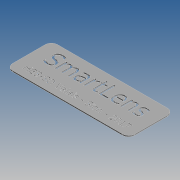
# Autodesk Inventor part: P306PlaqueLogo
Saved by Autodesk Inventor 2015 SP1 (Build 190203100, 203)
## iProperties
Created: 2017-01-31
Part Number: P306PlaqueLogo
Material: Générique
Document SubType Name: Modeling
Designer: serge.amoos
Density: 1 g/cm^3
Appearance: Par défaut
Author: serge.amoos
Autodesk Inventor part; units mm, degrees
ref_plane "YZ Plane" through (0, 0, 0) normal (1, 0, 0) x (0, 1, 0)
ref_plane "XZ Plane" through (0, 0, 0) normal (0, 1, 0) x (-1, 0, 0)
ref_plane "XY Plane" through (0, 0, 0) normal (0, 0, 1) x (1, 0, 0)
sketch "Sketch1" plane through (0, 0, 0) normal (0, 0, 1) x (1, 0, 0)
  line L0 (-27.65, 0) -> (27.65, 0) construction
  line L1 (0, -10.15) -> (0, 10.15) construction
  line L2 (-19.75, 7.25) -> (19.75, 7.25)
  line L3 (19.75, 7.25) -> (19.75, -7.25)
  line L4 (19.75, -7.25) -> (-19.75, -7.25)
  line L5 (-19.75, -7.25) -> (-19.75, 7.25)
  point P0 (0, 0)
  point P1 (0, 7.25)
  point P2 (19.75, 0)
  dimension "d0" = 39.5
  dimension "d1" = 14.5
  constraints: 8 end point, 2 midpoint, 2 parallel, 2 point on line, 1 horizontal, 1 perpendicular
  measures "d0" distance of L2.start L2.end
  measures "d1" distance of L2.end L3.end
extrude "Extrusion1" add sketch "Sketch1" along normal blind 0.4
fillet "Fillet1" radius 2 4 edges at (19.75, -7.25, 0.2) (19.75, 7.25, 0.2) (-19.75, 7.25, 0.2) (-19.75, -7.25, 0.2)
sketch "Sketch2" plane through (0, 0, 0.4) normal (0, 0, 1) x (1, 0, 0)
  line L0 (-29.6663, 8.3891) -> (29.6663, 8.3891) construction
  line L1 (29.6663, 8.3891) -> (29.6663, -8.3891) construction
  line L2 (29.6663, -8.3891) -> (-29.6663, -8.3891) construction
  line L3 (-29.6663, -8.3891) -> (-29.6663, 8.3891) construction
  line L4 (19.75, -5.25) -> (19.75, 5.25) projected
  line L5 (17.75, 7.25) -> (-17.75, 7.25) projected
  spline S0 degree 2 poles (-14.066, 0.0243) (-14.609, 0.0243) (-15.3707, 0.2512) (-15.707, 0.4133) knots 0 0 0 1 2 2 2
  line L6 (-15.707, 0.4133) -> (-15.707, 1.248)
  line L7 (-15.707, 1.248) -> (-15.6584, 1.248)
  spline S1 degree 2 poles (-15.6584, 1.248) (-15.3302, 0.94) (-14.4996, 0.5997) (-14.1147, 0.5997) knots 0 0 0 1 2 2 2
  spline S2 degree 2 poles (-14.1147, 0.5997) (-13.5636, 0.5997) (-13.0004, 1.0575) (-13.0004, 1.4343) knots 0 0 0 1 2 2 2
  spline S3 degree 2 poles (-13.0004, 1.4343) (-13.0004, 1.7342) (-13.2962, 2.1069) (-13.6163, 2.2001) knots 0 0 0 1 2 2 2
  spline S4 degree 2 poles (-13.6163, 2.2001) (-13.8472, 2.265) (-14.2322, 2.3541) (-14.5199, 2.427) knots 0 0 0 1 2 2 2
  spline S5 degree 2 poles (-14.5199, 2.427) (-14.7792, 2.4959) (-15.1884, 2.7026) (-15.3464, 2.8687) knots 0 0 0 1 2 2 2
  spline S6 degree 2 poles (-15.3464, 2.8687) (-15.5004, 3.0348) (-15.6706, 3.4805) (-15.6706, 3.7723) knots 0 0 0 1 2 2 2
  spline S7 degree 2 poles (-15.6706, 3.7723) (-15.6706, 4.38) (-14.7224, 5.2026) (-13.9891, 5.2026) knots 0 0 0 1 2 2 2
  spline S8 degree 2 poles (-13.9891, 5.2026) (-13.5677, 5.2026) (-12.8221, 5.0364) (-12.502, 4.8784) knots 0 0 0 1 2 2 2
  line L8 (-12.502, 4.8784) -> (-12.502, 4.0843)
  line L9 (-12.502, 4.0843) -> (-12.5506, 4.0843)
  spline S9 degree 2 poles (-12.5506, 4.0843) (-12.7897, 4.3031) (-13.5353, 4.6272) (-13.9445, 4.6272) knots 0 0 0 1 2 2 2
  spline S10 degree 2 poles (-13.9445, 4.6272) (-14.4064, 4.6272) (-14.9777, 4.1937) (-14.9777, 3.8411) knots 0 0 0 1 2 2 2
  spline S11 degree 2 poles (-14.9777, 3.8411) (-14.9777, 3.5251) (-14.6414, 3.1483) (-14.3254, 3.0632) knots 0 0 0 1 2 2 2
  spline S12 degree 2 poles (-14.3254, 3.0632) (-14.1147, 3.0065) (-13.5028, 2.8606) (-13.3002, 2.7998) knots 0 0 0 1 2 2 2
  spline S13 degree 2 poles (-13.3002, 2.7998) (-12.7857, 2.6418) (-12.3075, 2.0057) (-12.3075, 1.5397) knots 0 0 0 1 2 2 2
  spline S14 degree 2 poles (-12.3075, 1.5397) (-12.3075, 1.2439) (-12.5466, 0.6766) (-12.7613, 0.4781) knots 0 0 0 1 2 2 2
  spline S15 degree 2 poles (-12.7613, 0.4781) (-13.0004, 0.2593) (-13.6082, 0.0243) (-14.066, 0.0243) knots 0 0 0 1 2 2 2
  line L10 (-7.425, 0.1134) -> (-7.425, 2.2852)
  spline S16 degree 2 poles (-7.425, 2.2852) (-7.425, 2.5446) (-7.4656, 2.9862) (-7.5304, 3.1078) knots 0 0 0 1 2 2 2
  spline S17 degree 2 poles (-7.5304, 3.1078) (-7.5952, 3.2415) (-7.8424, 3.3711) (-8.0571, 3.3711) knots 0 0 0 1 2 2 2
  spline S18 degree 2 poles (-8.0571, 3.3711) (-8.2516, 3.3711) (-8.6973, 3.1321) (-8.9323, 2.9052) knots 0 0 0 1 2 2 2
  spline S19 degree 2 poles (-8.9323, 2.9052) (-8.9283, 2.8484) (-8.9202, 2.6904) (-8.9202, 2.5851) knots 0 0 0 1 2 2 2
  line L11 (-8.9202, 2.5851) -> (-8.9202, 0.1134)
  line L12 (-8.9202, 0.1134) -> (-9.5523, 0.1134)
  line L13 (-9.5523, 0.1134) -> (-9.5523, 2.2852)
  spline S20 degree 2 poles (-9.5523, 2.2852) (-9.5523, 2.5446) (-9.5928, 2.9862) (-9.6576, 3.1078) knots 0 0 0 1 2 2 2
  spline S21 degree 2 poles (-9.6576, 3.1078) (-9.7224, 3.2415) (-9.9696, 3.3711) (-10.1844, 3.3711) knots 0 0 0 1 2 2 2
  spline S22 degree 2 poles (-10.1844, 3.3711) (-10.387, 3.3711) (-10.8367, 3.1159) (-11.0474, 2.9173) knots 0 0 0 1 2 2 2
  line L14 (-11.0474, 2.9173) -> (-11.0474, 0.1134)
  line L15 (-11.0474, 0.1134) -> (-11.6795, 0.1134)
  line L16 (-11.6795, 0.1134) -> (-11.6795, 3.8655)
  line L17 (-11.6795, 3.8655) -> (-11.0474, 3.8655)
  line L18 (-11.0474, 3.8655) -> (-11.0474, 3.4522)
  spline S23 degree 2 poles (-11.0474, 3.4522) (-10.8002, 3.6993) (-10.314, 3.9708) (-10.0223, 3.9708) knots 0 0 0 1 2 2 2
  spline S24 degree 2 poles (-10.0223, 3.9708) (-9.69, 3.9708) (-9.1754, 3.6669) (-9.0417, 3.3225) knots 0 0 0 1 2 2 2
  spline S25 degree 2 poles (-9.0417, 3.3225) (-8.7541, 3.6426) (-8.2111, 3.9708) (-7.8951, 3.9708) knots 0 0 0 1 2 2 2
  spline S26 degree 2 poles (-7.8951, 3.9708) (-7.6519, 3.9708) (-7.2549, 3.8209) (-7.109, 3.6507) knots 0 0 0 1 2 2 2
  spline S27 degree 2 poles (-7.109, 3.6507) (-6.9591, 3.4805) (-6.7929, 2.97) (-6.7929, 2.5851) knots 0 0 0 1 2 2 2
  line L19 (-6.7929, 2.5851) -> (-6.7929, 0.1134)
  line L20 (-6.7929, 0.1134) -> (-7.425, 0.1134)
  spline S28 degree 2 poles (-3.8148, 0.5105) (-3.8918, 0.4538) (-4.1511, 0.2512) (-4.2727, 0.1904) knots 0 0 0 1 2 2 2
  spline S29 degree 2 poles (-4.2727, 0.1904) (-4.4388, 0.1013) (-4.7508, 0.0081) (-5.0344, 0.0081) knots 0 0 0 1 2 2 2
  spline S30 degree 2 poles (-5.0344, 0.0081) (-5.2654, 0.0081) (-5.6827, 0.1823) (-5.8408, 0.3403) knots 0 0 0 1 2 2 2
  spline S31 degree 2 poles (-5.8408, 0.3403) (-5.9907, 0.4943) (-6.173, 0.9481) (-6.173, 1.1993) knots 0 0 0 1 2 2 2
  spline S32 degree 2 poles (-6.173, 1.1993) (-6.173, 1.5883) (-5.8448, 2.1394) (-5.4882, 2.2974) knots 0 0 0 1 2 2 2
  spline S33 degree 2 poles (-5.4882, 2.2974) (-5.1722, 2.4433) (-4.3132, 2.5527) (-3.8148, 2.581) knots 0 0 0 1 2 2 2
  line L21 (-3.8148, 2.581) -> (-3.8148, 2.7026)
  spline S34 degree 2 poles (-3.8148, 2.7026) (-3.8148, 2.9214) (-3.9485, 3.1928) (-4.0701, 3.2698) knots 0 0 0 1 2 2 2
  spline S35 degree 2 poles (-4.0701, 3.2698) (-4.1917, 3.3468) (-4.5401, 3.3954) (-4.7265, 3.3954) knots 0 0 0 1 2 2 2
  spline S36 degree 2 poles (-4.7265, 3.3954) (-4.9453, 3.3954) (-5.5369, 3.2658) (-5.8327, 3.1402) knots 0 0 0 1 2 2 2
  line L22 (-5.8327, 3.1402) -> (-5.8691, 3.1402)
  line L23 (-5.8691, 3.1402) -> (-5.8691, 3.7844)
  spline S37 degree 2 poles (-5.8691, 3.7844) (-5.6949, 3.833) (-5.0425, 3.9546) (-4.7224, 3.9546) knots 0 0 0 1 2 2 2
  spline S38 degree 2 poles (-4.7224, 3.9546) (-4.3335, 3.9546) (-3.8027, 3.833) (-3.592, 3.675) knots 0 0 0 1 2 2 2
  spline S39 degree 2 poles (-3.592, 3.675) (-3.3853, 3.5211) (-3.1827, 3.0308) (-3.1827, 2.6783) knots 0 0 0 1 2 2 2
  line L24 (-3.1827, 2.6783) -> (-3.1827, 0.1134)
  line L25 (-3.1827, 0.1134) -> (-3.8148, 0.1134)
  line L26 (-3.8148, 0.1134) -> (-3.8148, 0.5105)
  line L27 (-3.8148, 1.0373) -> (-3.8148, 2.0786)
  spline S40 degree 2 poles (-3.8148, 2.0786) (-4.0417, 2.0583) (-4.7265, 1.9894) (-4.9412, 1.9246) knots 0 0 0 1 2 2 2
  spline S41 degree 2 poles (-4.9412, 1.9246) (-5.1925, 1.8476) (-5.5207, 1.5275) (-5.5207, 1.2439) knots 0 0 0 1 2 2 2
  spline S42 degree 2 poles (-5.5207, 1.2439) (-5.5207, 0.9198) (-5.156, 0.5916) (-4.8075, 0.5916) knots 0 0 0 1 2 2 2
  spline S43 degree 2 poles (-4.8075, 0.5916) (-4.5117, 0.5916) (-4.0255, 0.8468) (-3.8148, 1.0373) knots 0 0 0 1 2 2 2
  line L28 (-0.3059, 3.1888) -> (-0.3383, 3.1888)
  spline S44 degree 2 poles (-0.3383, 3.1888) (-0.4113, 3.2091) (-0.5693, 3.2172) (-0.6787, 3.2172) knots 0 0 0 1 2 2 2
  spline S45 degree 2 poles (-0.6787, 3.2172) (-0.934, 3.2172) (-1.4364, 2.9943) (-1.6633, 2.7755) knots 0 0 0 1 2 2 2
  line L29 (-1.6633, 2.7755) -> (-1.6633, 0.1134)
  line L30 (-1.6633, 0.1134) -> (-2.2954, 0.1134)
  line L31 (-2.2954, 0.1134) -> (-2.2954, 3.8655)
  line L32 (-2.2954, 3.8655) -> (-1.6633, 3.8655)
  line L33 (-1.6633, 3.8655) -> (-1.6633, 3.3063)
  spline S46 degree 2 poles (-1.6633, 3.3063) (-1.3189, 3.6142) (-0.8043, 3.8655) (-0.5612, 3.8655) knots 0 0 0 1 2 2 2
  spline S47 degree 2 poles (-0.5612, 3.8655) (-0.4639, 3.8655) (-0.3667, 3.8574) (-0.3059, 3.8452) knots 0 0 0 1 2 2 2
  line L34 (-0.3059, 3.8452) -> (-0.3059, 3.1888)
  spline S48 degree 2 poles (1.3189, 0.0405) (0.8043, 0.0405) (0.2249, 0.628) (0.2249, 1.2642) knots 0 0 0 1 2 2 2
  line L35 (0.2249, 1.2642) -> (0.2249, 3.3428)
  line L36 (0.2249, 3.3428) -> (-0.2006, 3.3428)
  line L37 (-0.2006, 3.3428) -> (-0.2006, 3.8655)
  line L38 (-0.2006, 3.8655) -> (0.2249, 3.8655)
  line L39 (0.2249, 3.8655) -> (0.2249, 4.9433)
  line L40 (0.2249, 4.9433) -> (0.857, 4.9433)
  line L41 (0.857, 4.9433) -> (0.857, 3.8655)
  line L42 (0.857, 3.8655) -> (2.0199, 3.8655)
  line L43 (2.0199, 3.8655) -> (2.0199, 3.3428)
  line L44 (2.0199, 3.3428) -> (0.857, 3.3428)
  line L45 (0.857, 3.3428) -> (0.857, 1.5559)
  spline S49 degree 2 poles (0.857, 1.5559) (0.857, 1.2723) (0.8772, 0.9603) (0.9461, 0.8266) knots 0 0 0 1 2 2 2
  spline S50 degree 2 poles (0.9461, 0.8266) (1.0028, 0.7091) (1.2581, 0.5916) (1.4769, 0.5916) knots 0 0 0 1 2 2 2
  spline S51 degree 2 poles (1.4769, 0.5916) (1.6309, 0.5916) (1.9186, 0.6847) (1.9834, 0.7131) knots 0 0 0 1 2 2 2
  line L46 (1.9834, 0.7131) -> (2.0199, 0.7131)
  line L47 (2.0199, 0.7131) -> (2.0199, 0.1458)
  spline S52 degree 2 poles (2.0199, 0.1458) (1.8416, 0.0972) (1.4769, 0.0405) (1.3189, 0.0405) knots 0 0 0 1 2 2 2
  line L48 (5.4315, 0.1134) -> (2.5344, 0.1134)
  line L49 (2.5344, 0.1134) -> (2.5344, 5.1134)
  line L50 (2.5344, 5.1134) -> (3.1989, 5.1134)
  line L51 (3.1989, 5.1134) -> (3.1989, 0.705)
  line L52 (3.1989, 0.705) -> (5.4315, 0.705)
  line L53 (5.4315, 0.705) -> (5.4315, 0.1134)
  spline S53 degree 2 poles (7.5344, 0.0283) (6.6349, 0.0283) (5.6463, 1.0373) (5.6463, 1.9692) knots 0 0 0 1 2 2 2
  spline S54 degree 2 poles (5.6463, 1.9692) (5.6463, 2.8849) (6.6066, 3.9708) (7.3805, 3.9708) knots 0 0 0 1 2 2 2
  spline S55 degree 2 poles (7.3805, 3.9708) (7.7289, 3.9708) (8.2678, 3.7682) (8.4664, 3.5535) knots 0 0 0 1 2 2 2
  spline S56 degree 2 poles (8.4664, 3.5535) (8.669, 3.3387) (8.8837, 2.7188) (8.8837, 2.269) knots 0 0 0 1 2 2 2
  line L54 (8.8837, 2.269) -> (8.8837, 1.9246)
  line L55 (8.8837, 1.9246) -> (6.2865, 1.9246)
  spline S57 degree 2 poles (6.2865, 1.9246) (6.2865, 1.2723) (6.9429, 0.5794) (7.5263, 0.5794) knots 0 0 0 1 2 2 2
  spline S58 degree 2 poles (7.5263, 0.5794) (7.733, 0.5794) (8.1341, 0.6726) (8.2962, 0.7455) knots 0 0 0 1 2 2 2
  spline S59 degree 2 poles (8.2962, 0.7455) (8.4664, 0.8266) (8.7014, 0.9684) (8.7784, 1.0332) knots 0 0 0 1 2 2 2
  line L56 (8.7784, 1.0332) -> (8.8148, 1.0332)
  line L57 (8.8148, 1.0332) -> (8.8148, 0.3444)
  spline S60 degree 2 poles (8.8148, 0.3444) (8.7054, 0.2998) (8.3732, 0.1702) (8.2435, 0.1337) knots 0 0 0 1 2 2 2
  spline S61 degree 2 poles (8.2435, 0.1337) (8.0612, 0.081) (7.7613, 0.0283) (7.5344, 0.0283) knots 0 0 0 1 2 2 2
  spline S62 degree 2 poles (8.2678, 2.4068) (8.2597, 2.6621) (8.1544, 3.0348) (8.0531, 3.1604) knots 0 0 0 1 2 2 2
  spline S63 degree 2 poles (8.0531, 3.1604) (7.9437, 3.3022) (7.5993, 3.4522) (7.344, 3.4522) knots 0 0 0 1 2 2 2
  spline S64 degree 2 poles (7.344, 3.4522) (7.0928, 3.4522) (6.7403, 3.3022) (6.5944, 3.1564) knots 0 0 0 1 2 2 2
  spline S65 degree 2 poles (6.5944, 3.1564) (6.4526, 3.0065) (6.3067, 2.6458) (6.2865, 2.4068) knots 0 0 0 1 2 2 2
  line L58 (6.2865, 2.4068) -> (8.2678, 2.4068)
  line L59 (12.4696, 0.1134) -> (11.8375, 0.1134)
  line L60 (11.8375, 0.1134) -> (11.8375, 2.2528)
  spline S66 degree 2 poles (11.8375, 2.2528) (11.8375, 2.5121) (11.7889, 2.9578) (11.716, 3.0916) knots 0 0 0 1 2 2 2
  spline S67 degree 2 poles (11.716, 3.0916) (11.639, 3.2334) (11.3635, 3.3711) (11.1284, 3.3711) knots 0 0 0 1 2 2 2
  spline S68 degree 2 poles (11.1284, 3.3711) (10.8934, 3.3711) (10.3951, 3.1199) (10.156, 2.9173) knots 0 0 0 1 2 2 2
  line L61 (10.156, 2.9173) -> (10.156, 0.1134)
  line L62 (10.156, 0.1134) -> (9.5239, 0.1134)
  line L63 (9.5239, 0.1134) -> (9.5239, 3.8655)
  line L64 (9.5239, 3.8655) -> (10.156, 3.8655)
  line L65 (10.156, 3.8655) -> (10.156, 3.4481)
  spline S69 degree 2 poles (10.156, 3.4481) (10.4396, 3.7034) (10.9866, 3.9708) (11.2946, 3.9708) knots 0 0 0 1 2 2 2
  spline S70 degree 2 poles (11.2946, 3.9708) (11.8456, 3.9708) (12.4696, 3.2415) (12.4696, 2.5486) knots 0 0 0 1 2 2 2
  line L66 (12.4696, 2.5486) -> (12.4696, 0.1134)
  spline S71 degree 2 poles (14.3699, 0.0243) (13.9931, 0.0243) (13.3408, 0.2269) (13.126, 0.3403) knots 0 0 0 1 2 2 2
  line L67 (13.126, 0.3403) -> (13.126, 1.0494)
  line L68 (13.126, 1.0494) -> (13.1584, 1.0494)
  spline S72 degree 2 poles (13.1584, 1.0494) (13.2395, 0.9846) (13.4583, 0.8306) (13.6406, 0.7455) knots 0 0 0 1 2 2 2
  spline S73 degree 2 poles (13.6406, 0.7455) (13.7986, 0.6685) (14.1876, 0.5551) (14.3942, 0.5551) knots 0 0 0 1 2 2 2
  spline S74 degree 2 poles (14.3942, 0.5551) (14.5442, 0.5551) (14.8886, 0.624) (14.9696, 0.6807) knots 0 0 0 1 2 2 2
  spline S75 degree 2 poles (14.9696, 0.6807) (15.0871, 0.7577) (15.1925, 0.9319) (15.1925, 1.1102) knots 0 0 0 1 2 2 2
  spline S76 degree 2 poles (15.1925, 1.1102) (15.1925, 1.333) (14.9494, 1.564) (14.6374, 1.641) knots 0 0 0 1 2 2 2
  spline S77 degree 2 poles (14.6374, 1.641) (14.5158, 1.6693) (14.1268, 1.7504) (13.9607, 1.795) knots 0 0 0 1 2 2 2
  spline S78 degree 2 poles (13.9607, 1.795) (13.5312, 1.9206) (13.1422, 2.4392) (13.1422, 2.8079) knots 0 0 0 1 2 2 2
  spline S79 degree 2 poles (13.1422, 2.8079) (13.1422, 3.3185) (13.908, 3.9546) (14.5401, 3.9546) knots 0 0 0 1 2 2 2
  spline S80 degree 2 poles (14.5401, 3.9546) (14.8521, 3.9546) (15.4842, 3.8006) (15.6989, 3.6831) knots 0 0 0 1 2 2 2
  line L69 (15.6989, 3.6831) -> (15.6989, 3.0065)
  line L70 (15.6989, 3.0065) -> (15.6665, 3.0065)
  spline S81 degree 2 poles (15.6665, 3.0065) (15.4234, 3.201) (14.8318, 3.4238) (14.528, 3.4238) knots 0 0 0 1 2 2 2
  spline S82 degree 2 poles (14.528, 3.4238) (14.216, 3.4238) (13.7865, 3.1604) (13.7865, 2.8971) knots 0 0 0 1 2 2 2
  spline S83 degree 2 poles (13.7865, 2.8971) (13.7865, 2.658) (14.0417, 2.427) (14.3254, 2.3541) knots 0 0 0 1 2 2 2
  spline S84 degree 2 poles (14.3254, 2.3541) (14.4631, 2.3176) (14.8116, 2.2447) (15.002, 2.2001) knots 0 0 0 1 2 2 2
  spline S85 degree 2 poles (15.002, 2.2001) (15.4153, 2.0948) (15.8367, 1.6126) (15.8367, 1.1953) knots 0 0 0 1 2 2 2
  spline S86 degree 2 poles (15.8367, 1.1953) (15.8367, 0.9522) (15.6463, 0.5227) (15.4599, 0.3646) knots 0 0 0 1 2 2 2
  spline S87 degree 2 poles (15.4599, 0.3646) (15.2613, 0.1985) (14.7549, 0.0243) (14.3699, 0.0243) knots 0 0 0 1 2 2 2
  line L71 (-15.2974, -5.1604) -> (-15.5632, -5.1604)
  line L72 (-15.5632, -5.1604) -> (-15.5632, -4.1815)
  line L73 (-15.5632, -4.1815) -> (-16.4838, -4.1815)
  line L74 (-16.4838, -4.1815) -> (-16.4838, -5.1604)
  line L75 (-16.4838, -5.1604) -> (-16.7496, -5.1604)
  line L76 (-16.7496, -5.1604) -> (-16.7496, -3.1604)
  line L77 (-16.7496, -3.1604) -> (-16.4838, -3.1604)
  line L78 (-16.4838, -3.1604) -> (-16.4838, -3.9449)
  line L79 (-16.4838, -3.9449) -> (-15.5632, -3.9449)
  line L80 (-15.5632, -3.9449) -> (-15.5632, -3.1604)
  line L81 (-15.5632, -3.1604) -> (-15.2974, -3.1604)
  line L82 (-15.2974, -3.1604) -> (-15.2974, -5.1604)
  line L83 (-14.8922, -5.1604) -> (-14.8922, -3.1604)
  line L84 (-14.8922, -3.1604) -> (-13.641, -3.1604)
  line L85 (-13.641, -3.1604) -> (-13.641, -3.3971)
  line L86 (-13.641, -3.3971) -> (-14.6264, -3.3971)
  line L87 (-14.6264, -3.3971) -> (-14.6264, -3.9449)
  line L88 (-14.6264, -3.9449) -> (-13.7075, -3.9449)
  line L89 (-13.7075, -3.9449) -> (-13.7075, -4.1815)
  line L90 (-13.7075, -4.1815) -> (-14.6264, -4.1815)
  line L91 (-14.6264, -4.1815) -> (-14.6264, -4.9238)
  line L92 (-14.6264, -4.9238) -> (-13.641, -4.9238)
  line L93 (-13.641, -4.9238) -> (-13.641, -5.1604)
  line L94 (-13.641, -5.1604) -> (-14.8922, -5.1604)
  spline S88 degree 2 poles (-12.7917, -5.1961) (-13.0089, -5.1961) (-13.3136, -5.1053) (-13.4481, -5.0405) knots 0 0 0 1 2 2 2
  line L95 (-13.4481, -5.0405) -> (-13.4481, -4.7066)
  line L96 (-13.4481, -4.7066) -> (-13.4287, -4.7066)
  spline S89 degree 2 poles (-13.4287, -4.7066) (-13.2974, -4.8298) (-12.9652, -4.9659) (-12.8112, -4.9659) knots 0 0 0 1 2 2 2
  spline S90 degree 2 poles (-12.8112, -4.9659) (-12.5908, -4.9659) (-12.3655, -4.7828) (-12.3655, -4.6321) knots 0 0 0 1 2 2 2
  spline S91 degree 2 poles (-12.3655, -4.6321) (-12.3655, -4.5121) (-12.4838, -4.363) (-12.6118, -4.3258) knots 0 0 0 1 2 2 2
  spline S92 degree 2 poles (-12.6118, -4.3258) (-12.7042, -4.2998) (-12.8582, -4.2642) (-12.9733, -4.235) knots 0 0 0 1 2 2 2
  spline S93 degree 2 poles (-12.9733, -4.235) (-13.077, -4.2074) (-13.2407, -4.1248) (-13.3039, -4.0583) knots 0 0 0 1 2 2 2
  spline S94 degree 2 poles (-13.3039, -4.0583) (-13.3655, -3.9919) (-13.4336, -3.8136) (-13.4336, -3.6969) knots 0 0 0 1 2 2 2
  spline S95 degree 2 poles (-13.4336, -3.6969) (-13.4336, -3.4538) (-13.0543, -3.1248) (-12.7609, -3.1248) knots 0 0 0 1 2 2 2
  spline S96 degree 2 poles (-12.7609, -3.1248) (-12.5924, -3.1248) (-12.2942, -3.1912) (-12.1661, -3.2544) knots 0 0 0 1 2 2 2
  line L97 (-12.1661, -3.2544) -> (-12.1661, -3.5721)
  line L98 (-12.1661, -3.5721) -> (-12.1856, -3.5721)
  spline S97 degree 2 poles (-12.1856, -3.5721) (-12.2812, -3.4846) (-12.5794, -3.3549) (-12.7431, -3.3549) knots 0 0 0 1 2 2 2
  spline S98 degree 2 poles (-12.7431, -3.3549) (-12.9279, -3.3549) (-13.1564, -3.5283) (-13.1564, -3.6693) knots 0 0 0 1 2 2 2
  spline S99 degree 2 poles (-13.1564, -3.6693) (-13.1564, -3.7958) (-13.0219, -3.9465) (-12.8955, -3.9805) knots 0 0 0 1 2 2 2
  spline S100 degree 2 poles (-12.8955, -3.9805) (-12.8112, -4.0032) (-12.5665, -4.0616) (-12.4854, -4.0859) knots 0 0 0 1 2 2 2
  spline S101 degree 2 poles (-12.4854, -4.0859) (-12.2796, -4.1491) (-12.0883, -4.4035) (-12.0883, -4.5899) knots 0 0 0 1 2 2 2
  spline S102 degree 2 poles (-12.0883, -4.5899) (-12.0883, -4.7082) (-12.184, -4.9352) (-12.2699, -5.0146) knots 0 0 0 1 2 2 2
  spline S103 degree 2 poles (-12.2699, -5.0146) (-12.3655, -5.1021) (-12.6086, -5.1961) (-12.7917, -5.1961) knots 0 0 0 1 2 2 2
  line L99 (-11.1418, -4.4068) -> (-11.8987, -4.4068)
  line L100 (-11.8987, -4.4068) -> (-11.8987, -4.1637)
  line L101 (-11.8987, -4.1637) -> (-11.1418, -4.1637)
  line L102 (-11.1418, -4.1637) -> (-11.1418, -4.4068)
  spline S104 degree 2 poles (-10.2618, -5.1961) (-10.4789, -5.1961) (-10.7836, -5.1053) (-10.9182, -5.0405) knots 0 0 0 1 2 2 2
  line L103 (-10.9182, -5.0405) -> (-10.9182, -4.7066)
  line L104 (-10.9182, -4.7066) -> (-10.8987, -4.7066)
  spline S105 degree 2 poles (-10.8987, -4.7066) (-10.7674, -4.8298) (-10.4352, -4.9659) (-10.2812, -4.9659) knots 0 0 0 1 2 2 2
  spline S106 degree 2 poles (-10.2812, -4.9659) (-10.0608, -4.9659) (-9.8355, -4.7828) (-9.8355, -4.6321) knots 0 0 0 1 2 2 2
  spline S107 degree 2 poles (-9.8355, -4.6321) (-9.8355, -4.5121) (-9.9538, -4.363) (-10.0818, -4.3258) knots 0 0 0 1 2 2 2
  spline S108 degree 2 poles (-10.0818, -4.3258) (-10.1742, -4.2998) (-10.3282, -4.2642) (-10.4433, -4.235) knots 0 0 0 1 2 2 2
  spline S109 degree 2 poles (-10.4433, -4.235) (-10.547, -4.2074) (-10.7107, -4.1248) (-10.7739, -4.0583) knots 0 0 0 1 2 2 2
  spline S110 degree 2 poles (-10.7739, -4.0583) (-10.8355, -3.9919) (-10.9036, -3.8136) (-10.9036, -3.6969) knots 0 0 0 1 2 2 2
  spline S111 degree 2 poles (-10.9036, -3.6969) (-10.9036, -3.4538) (-10.5243, -3.1248) (-10.231, -3.1248) knots 0 0 0 1 2 2 2
  spline S112 degree 2 poles (-10.231, -3.1248) (-10.0624, -3.1248) (-9.7642, -3.1912) (-9.6361, -3.2544) knots 0 0 0 1 2 2 2
  line L105 (-9.6361, -3.2544) -> (-9.6361, -3.5721)
  line L106 (-9.6361, -3.5721) -> (-9.6556, -3.5721)
  spline S113 degree 2 poles (-9.6556, -3.5721) (-9.7512, -3.4846) (-10.0494, -3.3549) (-10.2131, -3.3549) knots 0 0 0 1 2 2 2
  spline S114 degree 2 poles (-10.2131, -3.3549) (-10.3979, -3.3549) (-10.6264, -3.5283) (-10.6264, -3.6693) knots 0 0 0 1 2 2 2
  spline S115 degree 2 poles (-10.6264, -3.6693) (-10.6264, -3.7958) (-10.4919, -3.9465) (-10.3655, -3.9805) knots 0 0 0 1 2 2 2
  spline S116 degree 2 poles (-10.3655, -3.9805) (-10.2812, -4.0032) (-10.0365, -4.0616) (-9.9554, -4.0859) knots 0 0 0 1 2 2 2
  spline S117 degree 2 poles (-9.9554, -4.0859) (-9.7496, -4.1491) (-9.5583, -4.4035) (-9.5583, -4.5899) knots 0 0 0 1 2 2 2
  spline S118 degree 2 poles (-9.5583, -4.5899) (-9.5583, -4.7082) (-9.654, -4.9352) (-9.7399, -5.0146) knots 0 0 0 1 2 2 2
  spline S119 degree 2 poles (-9.7399, -5.0146) (-9.8355, -5.1021) (-10.0786, -5.1961) (-10.2618, -5.1961) knots 0 0 0 1 2 2 2
  spline S120 degree 2 poles (-7.8728, -3.389) (-7.7593, -3.5219) (-7.6329, -3.9108) (-7.6329, -4.1604) knots 0 0 0 1 2 2 2
  spline S121 degree 2 poles (-7.6329, -4.1604) (-7.6329, -4.4035) (-7.7561, -4.7974) (-7.8728, -4.9303) knots 0 0 0 1 2 2 2
  spline S122 degree 2 poles (-7.8728, -4.9303) (-7.9959, -5.0697) (-8.3217, -5.2026) (-8.5178, -5.2026) knots 0 0 0 1 2 2 2
  spline S123 degree 2 poles (-8.5178, -5.2026) (-8.7204, -5.2026) (-9.0446, -5.0648) (-9.1629, -4.9303) knots 0 0 0 1 2 2 2
  spline S124 degree 2 poles (-9.1629, -4.9303) (-9.278, -4.7974) (-9.4011, -4.4068) (-9.4011, -4.1604) knots 0 0 0 1 2 2 2
  spline S125 degree 2 poles (-9.4011, -4.1604) (-9.4011, -3.9092) (-9.2763, -3.5267) (-9.1613, -3.389) knots 0 0 0 1 2 2 2
  spline S126 degree 2 poles (-9.1613, -3.389) (-9.0446, -3.2561) (-8.7188, -3.1183) (-8.5178, -3.1183) knots 0 0 0 1 2 2 2
  spline S127 degree 2 poles (-8.5178, -3.1183) (-8.3136, -3.1183) (-7.9862, -3.2609) (-7.8728, -3.389) knots 0 0 0 1 2 2 2
  spline S128 degree 2 poles (-7.91, -4.1604) (-7.91, -3.9627) (-7.9959, -3.6564) (-8.0737, -3.5559) knots 0 0 0 1 2 2 2
  spline S129 degree 2 poles (-8.0737, -3.5559) (-8.1532, -3.4522) (-8.3768, -3.3484) (-8.5162, -3.3484) knots 0 0 0 1 2 2 2
  spline S130 degree 2 poles (-8.5162, -3.3484) (-8.6605, -3.3484) (-8.8776, -3.4489) (-8.9603, -3.5559) knots 0 0 0 1 2 2 2
  spline S131 degree 2 poles (-8.9603, -3.5559) (-9.0397, -3.658) (-9.124, -3.9659) (-9.124, -4.1604) knots 0 0 0 1 2 2 2
  spline S132 degree 2 poles (-9.124, -4.1604) (-9.124, -4.5543) (-8.7934, -4.9724) (-8.5162, -4.9724) knots 0 0 0 1 2 2 2
  spline S133 degree 2 poles (-8.5162, -4.9724) (-8.2391, -4.9724) (-7.91, -4.5543) (-7.91, -4.1604) knots 0 0 0 1 2 2 2
  line L107 (-5.0316, -3.1604) -> (-5.7204, -5.1604)
  line L108 (-5.7204, -5.1604) -> (-6.0073, -5.1604)
  line L109 (-6.0073, -5.1604) -> (-6.6961, -3.1604)
  line L110 (-6.6961, -3.1604) -> (-6.4109, -3.1604)
  line L111 (-6.4109, -3.1604) -> (-5.8566, -4.8217)
  line L112 (-5.8566, -4.8217) -> (-5.3023, -3.1604)
  line L113 (-5.3023, -3.1604) -> (-5.0316, -3.1604)
  spline S134 degree 2 poles (-4.0235, -5.0016) (-4.0543, -5.0243) (-4.158, -5.1053) (-4.2066, -5.1296) knots 0 0 0 1 2 2 2
  spline S135 degree 2 poles (-4.2066, -5.1296) (-4.2731, -5.1653) (-4.3979, -5.2026) (-4.5113, -5.2026) knots 0 0 0 1 2 2 2
  spline S136 degree 2 poles (-4.5113, -5.2026) (-4.6037, -5.2026) (-4.7707, -5.1329) (-4.8339, -5.0697) knots 0 0 0 1 2 2 2
  spline S137 degree 2 poles (-4.8339, -5.0697) (-4.8938, -5.0081) (-4.9668, -4.8266) (-4.9668, -4.7261) knots 0 0 0 1 2 2 2
  spline S138 degree 2 poles (-4.9668, -4.7261) (-4.9668, -4.5705) (-4.8355, -4.3501) (-4.6929, -4.2869) knots 0 0 0 1 2 2 2
  spline S139 degree 2 poles (-4.6929, -4.2869) (-4.5665, -4.2285) (-4.2229, -4.1847) (-4.0235, -4.1734) knots 0 0 0 1 2 2 2
  line L114 (-4.0235, -4.1734) -> (-4.0235, -4.1248)
  spline S140 degree 2 poles (-4.0235, -4.1248) (-4.0235, -4.0373) (-4.077, -3.9287) (-4.1256, -3.8979) knots 0 0 0 1 2 2 2
  spline S141 degree 2 poles (-4.1256, -3.8979) (-4.1742, -3.8671) (-4.3136, -3.8476) (-4.3882, -3.8476) knots 0 0 0 1 2 2 2
  spline S142 degree 2 poles (-4.3882, -3.8476) (-4.4757, -3.8476) (-4.7123, -3.8995) (-4.8306, -3.9497) knots 0 0 0 1 2 2 2
  line L115 (-4.8306, -3.9497) -> (-4.8452, -3.9497)
  line L116 (-4.8452, -3.9497) -> (-4.8452, -3.692)
  spline S143 degree 2 poles (-4.8452, -3.692) (-4.7755, -3.6726) (-4.5146, -3.624) (-4.3865, -3.624) knots 0 0 0 1 2 2 2
  spline S144 degree 2 poles (-4.3865, -3.624) (-4.231, -3.624) (-4.0186, -3.6726) (-3.9344, -3.7358) knots 0 0 0 1 2 2 2
  spline S145 degree 2 poles (-3.9344, -3.7358) (-3.8517, -3.7974) (-3.7707, -3.9935) (-3.7707, -4.1345) knots 0 0 0 1 2 2 2
  line L117 (-3.7707, -4.1345) -> (-3.7707, -5.1604)
  line L118 (-3.7707, -5.1604) -> (-4.0235, -5.1604)
  line L119 (-4.0235, -5.1604) -> (-4.0235, -5.0016)
  line L120 (-4.0235, -4.7909) -> (-4.0235, -4.3744)
  spline S146 degree 2 poles (-4.0235, -4.3744) (-4.1143, -4.3825) (-4.3882, -4.41) (-4.4741, -4.436) knots 0 0 0 1 2 2 2
  spline S147 degree 2 poles (-4.4741, -4.436) (-4.5746, -4.4668) (-4.7058, -4.5948) (-4.7058, -4.7082) knots 0 0 0 1 2 2 2
  spline S148 degree 2 poles (-4.7058, -4.7082) (-4.7058, -4.8379) (-4.56, -4.9692) (-4.4206, -4.9692) knots 0 0 0 1 2 2 2
  spline S149 degree 2 poles (-4.4206, -4.9692) (-4.3023, -4.9692) (-4.1078, -4.8671) (-4.0235, -4.7909) knots 0 0 0 1 2 2 2
  line L121 (-3.158, -5.1604) -> (-3.4109, -5.1604)
  line L122 (-3.4109, -5.1604) -> (-3.4109, -3.0713)
  line L123 (-3.4109, -3.0713) -> (-3.158, -3.0713)
  line L124 (-3.158, -3.0713) -> (-3.158, -5.1604)
  spline S150 degree 2 poles (-1.9506, -5.0016) (-1.9814, -5.0243) (-2.0851, -5.1053) (-2.1337, -5.1296) knots 0 0 0 1 2 2 2
  spline S151 degree 2 poles (-2.1337, -5.1296) (-2.2002, -5.1653) (-2.325, -5.2026) (-2.4384, -5.2026) knots 0 0 0 1 2 2 2
  spline S152 degree 2 poles (-2.4384, -5.2026) (-2.5308, -5.2026) (-2.6977, -5.1329) (-2.7609, -5.0697) knots 0 0 0 1 2 2 2
  spline S153 degree 2 poles (-2.7609, -5.0697) (-2.8209, -5.0081) (-2.8938, -4.8266) (-2.8938, -4.7261) knots 0 0 0 1 2 2 2
  spline S154 degree 2 poles (-2.8938, -4.7261) (-2.8938, -4.5705) (-2.7626, -4.3501) (-2.6199, -4.2869) knots 0 0 0 1 2 2 2
  spline S155 degree 2 poles (-2.6199, -4.2869) (-2.4935, -4.2285) (-2.1499, -4.1847) (-1.9506, -4.1734) knots 0 0 0 1 2 2 2
  line L125 (-1.9506, -4.1734) -> (-1.9506, -4.1248)
  spline S156 degree 2 poles (-1.9506, -4.1248) (-1.9506, -4.0373) (-2.0041, -3.9287) (-2.0527, -3.8979) knots 0 0 0 1 2 2 2
  spline S157 degree 2 poles (-2.0527, -3.8979) (-2.1013, -3.8671) (-2.2407, -3.8476) (-2.3152, -3.8476) knots 0 0 0 1 2 2 2
  spline S158 degree 2 poles (-2.3152, -3.8476) (-2.4028, -3.8476) (-2.6394, -3.8995) (-2.7577, -3.9497) knots 0 0 0 1 2 2 2
  line L126 (-2.7577, -3.9497) -> (-2.7723, -3.9497)
  line L127 (-2.7723, -3.9497) -> (-2.7723, -3.692)
  spline S159 degree 2 poles (-2.7723, -3.692) (-2.7026, -3.6726) (-2.4417, -3.624) (-2.3136, -3.624) knots 0 0 0 1 2 2 2
  spline S160 degree 2 poles (-2.3136, -3.624) (-2.158, -3.624) (-1.9457, -3.6726) (-1.8614, -3.7358) knots 0 0 0 1 2 2 2
  spline S161 degree 2 poles (-1.8614, -3.7358) (-1.7788, -3.7974) (-1.6977, -3.9935) (-1.6977, -4.1345) knots 0 0 0 1 2 2 2
  line L128 (-1.6977, -4.1345) -> (-1.6977, -5.1604)
  line L129 (-1.6977, -5.1604) -> (-1.9506, -5.1604)
  line L130 (-1.9506, -5.1604) -> (-1.9506, -5.0016)
  line L131 (-1.9506, -4.7909) -> (-1.9506, -4.3744)
  spline S162 degree 2 poles (-1.9506, -4.3744) (-2.0413, -4.3825) (-2.3152, -4.41) (-2.4011, -4.436) knots 0 0 0 1 2 2 2
  spline S163 degree 2 poles (-2.4011, -4.436) (-2.5016, -4.4668) (-2.6329, -4.5948) (-2.6329, -4.7082) knots 0 0 0 1 2 2 2
  spline S164 degree 2 poles (-2.6329, -4.7082) (-2.6329, -4.8379) (-2.487, -4.9692) (-2.3477, -4.9692) knots 0 0 0 1 2 2 2
  spline S165 degree 2 poles (-2.3477, -4.9692) (-2.2293, -4.9692) (-2.0348, -4.8671) (-1.9506, -4.7909) knots 0 0 0 1 2 2 2
  line L132 (-1.0851, -5.1604) -> (-1.3379, -5.1604)
  line L133 (-1.3379, -5.1604) -> (-1.3379, -3.6596)
  line L134 (-1.3379, -3.6596) -> (-1.0851, -3.6596)
  line L135 (-1.0851, -3.6596) -> (-1.0851, -5.1604)
  line L136 (-1.0673, -3.41) -> (-1.3541, -3.41)
  line L137 (-1.3541, -3.41) -> (-1.3541, -3.1475)
  line L138 (-1.3541, -3.1475) -> (-1.0673, -3.1475)
  line L139 (-1.0673, -3.1475) -> (-1.0673, -3.41)
  spline S166 degree 2 poles (-0.3088, -5.1961) (-0.4595, -5.1961) (-0.7204, -5.1151) (-0.8063, -5.0697) knots 0 0 0 1 2 2 2
  line L140 (-0.8063, -5.0697) -> (-0.8063, -4.786)
  line L141 (-0.8063, -4.786) -> (-0.7934, -4.786)
  spline S167 degree 2 poles (-0.7934, -4.786) (-0.7609, -4.812) (-0.6734, -4.8736) (-0.6005, -4.9076) knots 0 0 0 1 2 2 2
  spline S168 degree 2 poles (-0.6005, -4.9076) (-0.5373, -4.9384) (-0.3817, -4.9838) (-0.299, -4.9838) knots 0 0 0 1 2 2 2
  spline S169 degree 2 poles (-0.299, -4.9838) (-0.2391, -4.9838) (-0.1013, -4.9562) (-0.0689, -4.9335) knots 0 0 0 1 2 2 2
  spline S170 degree 2 poles (-0.0689, -4.9335) (-0.0219, -4.9027) (0.0203, -4.833) (0.0203, -4.7617) knots 0 0 0 1 2 2 2
  spline S171 degree 2 poles (0.0203, -4.7617) (0.0203, -4.6726) (-0.077, -4.5802) (-0.2018, -4.5494) knots 0 0 0 1 2 2 2
  spline S172 degree 2 poles (-0.2018, -4.5494) (-0.2504, -4.5381) (-0.406, -4.5057) (-0.4724, -4.4878) knots 0 0 0 1 2 2 2
  spline S173 degree 2 poles (-0.4724, -4.4878) (-0.6442, -4.4376) (-0.7998, -4.2301) (-0.7998, -4.0826) knots 0 0 0 1 2 2 2
  spline S174 degree 2 poles (-0.7998, -4.0826) (-0.7998, -3.8784) (-0.4935, -3.624) (-0.2407, -3.624) knots 0 0 0 1 2 2 2
  spline S175 degree 2 poles (-0.2407, -3.624) (-0.1159, -3.624) (0.137, -3.6856) (0.2229, -3.7326) knots 0 0 0 1 2 2 2
  line L142 (0.2229, -3.7326) -> (0.2229, -4.0032)
  line L143 (0.2229, -4.0032) -> (0.2099, -4.0032)
  spline S176 degree 2 poles (0.2099, -4.0032) (0.1126, -3.9254) (-0.124, -3.8363) (-0.2455, -3.8363) knots 0 0 0 1 2 2 2
  spline S177 degree 2 poles (-0.2455, -3.8363) (-0.3703, -3.8363) (-0.5421, -3.9416) (-0.5421, -4.047) knots 0 0 0 1 2 2 2
  spline S178 degree 2 poles (-0.5421, -4.047) (-0.5421, -4.1426) (-0.44, -4.235) (-0.3266, -4.2642) knots 0 0 0 1 2 2 2
  spline S179 degree 2 poles (-0.3266, -4.2642) (-0.2715, -4.2787) (-0.1321, -4.3079) (-0.0559, -4.3258) knots 0 0 0 1 2 2 2
  spline S180 degree 2 poles (-0.0559, -4.3258) (0.1094, -4.3679) (0.278, -4.5608) (0.278, -4.7277) knots 0 0 0 1 2 2 2
  spline S181 degree 2 poles (0.278, -4.7277) (0.278, -4.8249) (0.2018, -4.9967) (0.1272, -5.0599) knots 0 0 0 1 2 2 2
  spline S182 degree 2 poles (0.1272, -5.0599) (0.0478, -5.1264) (-0.1548, -5.1961) (-0.3088, -5.1961) knots 0 0 0 1 2 2 2
  line L144 (2.0673, -4.4068) -> (1.3104, -4.4068)
  line L145 (1.3104, -4.4068) -> (1.3104, -4.1637)
  line L146 (1.3104, -4.1637) -> (2.0673, -4.1637)
  line L147 (2.0673, -4.1637) -> (2.0673, -4.4068)
  spline S183 degree 2 poles (3.8063, -5.1961) (3.5891, -5.1961) (3.2844, -5.1053) (3.1499, -5.0405) knots 0 0 0 1 2 2 2
  line L148 (3.1499, -5.0405) -> (3.1499, -4.7066)
  line L149 (3.1499, -4.7066) -> (3.1694, -4.7066)
  spline S184 degree 2 poles (3.1694, -4.7066) (3.3006, -4.8298) (3.6329, -4.9659) (3.7869, -4.9659) knots 0 0 0 1 2 2 2
  spline S185 degree 2 poles (3.7869, -4.9659) (4.0073, -4.9659) (4.2326, -4.7828) (4.2326, -4.6321) knots 0 0 0 1 2 2 2
  spline S186 degree 2 poles (4.2326, -4.6321) (4.2326, -4.5121) (4.1143, -4.363) (3.9862, -4.3258) knots 0 0 0 1 2 2 2
  spline S187 degree 2 poles (3.9862, -4.3258) (3.8938, -4.2998) (3.7399, -4.2642) (3.6248, -4.235) knots 0 0 0 1 2 2 2
  spline S188 degree 2 poles (3.6248, -4.235) (3.5211, -4.2074) (3.3574, -4.1248) (3.2942, -4.0583) knots 0 0 0 1 2 2 2
  spline S189 degree 2 poles (3.2942, -4.0583) (3.2326, -3.9919) (3.1645, -3.8136) (3.1645, -3.6969) knots 0 0 0 1 2 2 2
  spline S190 degree 2 poles (3.1645, -3.6969) (3.1645, -3.4538) (3.5438, -3.1248) (3.8371, -3.1248) knots 0 0 0 1 2 2 2
  spline S191 degree 2 poles (3.8371, -3.1248) (4.0057, -3.1248) (4.3039, -3.1912) (4.4319, -3.2544) knots 0 0 0 1 2 2 2
  line L150 (4.4319, -3.2544) -> (4.4319, -3.5721)
  line L151 (4.4319, -3.5721) -> (4.4125, -3.5721)
  spline S192 degree 2 poles (4.4125, -3.5721) (4.3169, -3.4846) (4.0186, -3.3549) (3.8549, -3.3549) knots 0 0 0 1 2 2 2
  spline S193 degree 2 poles (3.8549, -3.3549) (3.6702, -3.3549) (3.4417, -3.5283) (3.4417, -3.6693) knots 0 0 0 1 2 2 2
  spline S194 degree 2 poles (3.4417, -3.6693) (3.4417, -3.7958) (3.5762, -3.9465) (3.7026, -3.9805) knots 0 0 0 1 2 2 2
  spline S195 degree 2 poles (3.7026, -3.9805) (3.7869, -4.0032) (4.0316, -4.0616) (4.1126, -4.0859) knots 0 0 0 1 2 2 2
  spline S196 degree 2 poles (4.1126, -4.0859) (4.3185, -4.1491) (4.5097, -4.4035) (4.5097, -4.5899) knots 0 0 0 1 2 2 2
  spline S197 degree 2 poles (4.5097, -4.5899) (4.5097, -4.7082) (4.4141, -4.9352) (4.3282, -5.0146) knots 0 0 0 1 2 2 2
  spline S198 degree 2 poles (4.3282, -5.0146) (4.2326, -5.1021) (3.9895, -5.1961) (3.8063, -5.1961) knots 0 0 0 1 2 2 2
  line L152 (5.0186, -5.1604) -> (4.7658, -5.1604)
  line L153 (4.7658, -5.1604) -> (4.7658, -3.6596)
  line L154 (4.7658, -3.6596) -> (5.0186, -3.6596)
  line L155 (5.0186, -3.6596) -> (5.0186, -5.1604)
  line L156 (5.0365, -3.41) -> (4.7496, -3.41)
  line L157 (4.7496, -3.41) -> (4.7496, -3.1475)
  line L158 (4.7496, -3.1475) -> (5.0365, -3.1475)
  line L159 (5.0365, -3.1475) -> (5.0365, -3.41)
  spline S199 degree 2 poles (6.6232, -4.41) (6.6232, -4.7893) (6.2585, -5.2026) (5.9538, -5.2026) knots 0 0 0 1 2 2 2
  spline S200 degree 2 poles (5.9538, -5.2026) (5.641, -5.2026) (5.2828, -4.7763) (5.2828, -4.41) knots 0 0 0 1 2 2 2
  spline S201 degree 2 poles (5.2828, -4.41) (5.2828, -4.034) (5.6523, -3.6175) (5.9538, -3.6175) knots 0 0 0 1 2 2 2
  spline S202 degree 2 poles (5.9538, -3.6175) (6.2585, -3.6175) (6.6232, -4.0324) (6.6232, -4.41) knots 0 0 0 1 2 2 2
  spline S203 degree 2 poles (6.3622, -4.41) (6.3622, -4.1183) (6.1499, -3.8347) (5.9538, -3.8347) knots 0 0 0 1 2 2 2
  spline S204 degree 2 poles (5.9538, -3.8347) (5.7577, -3.8347) (5.5438, -4.1183) (5.5438, -4.41) knots 0 0 0 1 2 2 2
  spline S205 degree 2 poles (5.5438, -4.41) (5.5438, -4.6937) (5.7577, -4.9854) (5.9538, -4.9854) knots 0 0 0 1 2 2 2
  spline S206 degree 2 poles (5.9538, -4.9854) (6.1483, -4.9854) (6.3622, -4.6985) (6.3622, -4.41) knots 0 0 0 1 2 2 2
  line L160 (8.0608, -5.1604) -> (7.8079, -5.1604)
  line L161 (7.8079, -5.1604) -> (7.8079, -4.3047)
  spline S207 degree 2 poles (7.8079, -4.3047) (7.8079, -4.201) (7.7885, -4.0227) (7.7593, -3.9692) knots 0 0 0 1 2 2 2
  spline S208 degree 2 poles (7.7593, -3.9692) (7.7285, -3.9125) (7.6183, -3.8574) (7.5243, -3.8574) knots 0 0 0 1 2 2 2
  spline S209 degree 2 poles (7.5243, -3.8574) (7.4303, -3.8574) (7.231, -3.9578) (7.1353, -4.0389) knots 0 0 0 1 2 2 2
  line L162 (7.1353, -4.0389) -> (7.1353, -5.1604)
  line L163 (7.1353, -5.1604) -> (6.8825, -5.1604)
  line L164 (6.8825, -5.1604) -> (6.8825, -3.6596)
  line L165 (6.8825, -3.6596) -> (7.1353, -3.6596)
  line L166 (7.1353, -3.6596) -> (7.1353, -3.8266)
  spline S210 degree 2 poles (7.1353, -3.8266) (7.2488, -3.7245) (7.4676, -3.6175) (7.5908, -3.6175) knots 0 0 0 1 2 2 2
  spline S211 degree 2 poles (7.5908, -3.6175) (7.8112, -3.6175) (8.0608, -3.9092) (8.0608, -4.1864) knots 0 0 0 1 2 2 2
  line L167 (8.0608, -4.1864) -> (8.0608, -5.1604)
  line L168 (9.97, -4.4068) -> (9.2131, -4.4068)
  line L169 (9.2131, -4.4068) -> (9.2131, -4.1637)
  line L170 (9.2131, -4.1637) -> (9.97, -4.1637)
  line L171 (9.97, -4.1637) -> (9.97, -4.4068)
  line L172 (12.3282, -5.1604) -> (11.0948, -5.1604)
  line L173 (11.0948, -5.1604) -> (11.0948, -4.8768)
  spline S212 degree 2 poles (11.0948, -4.8768) (11.2277, -4.752) (11.4643, -4.5202) (11.5778, -4.3954) knots 0 0 0 1 2 2 2
  spline S213 degree 2 poles (11.5778, -4.3954) (11.8063, -4.1442) (11.9733, -3.8428) (11.9733, -3.6823) knots 0 0 0 1 2 2 2
  spline S214 degree 2 poles (11.9733, -3.6823) (11.9733, -3.598) (11.9214, -3.4716) (11.8744, -3.4311) knots 0 0 0 1 2 2 2
  spline S215 degree 2 poles (11.8744, -3.4311) (11.8274, -3.3906) (11.7042, -3.3501) (11.6297, -3.3501) knots 0 0 0 1 2 2 2
  spline S216 degree 2 poles (11.6297, -3.3501) (11.5583, -3.3501) (11.4125, -3.3857) (11.346, -3.4133) knots 0 0 0 1 2 2 2
  spline S217 degree 2 poles (11.346, -3.4133) (11.2893, -3.436) (11.184, -3.5008) (11.1515, -3.5235) knots 0 0 0 1 2 2 2
  line L174 (11.1515, -3.5235) -> (11.137, -3.5235)
  line L175 (11.137, -3.5235) -> (11.137, -3.2382)
  spline S218 degree 2 poles (11.137, -3.2382) (11.2196, -3.1977) (11.5162, -3.1183) (11.6491, -3.1183) knots 0 0 0 1 2 2 2
  spline S219 degree 2 poles (11.6491, -3.1183) (11.9295, -3.1183) (12.2455, -3.4149) (12.2455, -3.6677) knots 0 0 0 1 2 2 2
  spline S220 degree 2 poles (12.2455, -3.6677) (12.2455, -3.786) (12.1904, -3.9838) (12.1418, -4.0681) knots 0 0 0 1 2 2 2
  spline S221 degree 2 poles (12.1418, -4.0681) (12.0932, -4.1556) (11.9522, -4.3274) (11.8744, -4.41) knots 0 0 0 1 2 2 2
  spline S222 degree 2 poles (11.8744, -4.41) (11.748, -4.5478) (11.4384, -4.8428) (11.346, -4.9287) knots 0 0 0 1 2 2 2
  line L176 (11.346, -4.9287) -> (12.3282, -4.9287)
  line L177 (12.3282, -4.9287) -> (12.3282, -5.1604)
  spline S223 degree 2 poles (13.8404, -4.1604) (13.8404, -4.6985) (13.5276, -5.2026) (13.2018, -5.2026) knots 0 0 0 1 2 2 2
  spline S224 degree 2 poles (13.2018, -5.2026) (12.8711, -5.2026) (12.5616, -4.6888) (12.5616, -4.1621) knots 0 0 0 1 2 2 2
  spline S225 degree 2 poles (12.5616, -4.1621) (12.5616, -3.6207) (12.8744, -3.1199) (13.2018, -3.1199) knots 0 0 0 1 2 2 2
  spline S226 degree 2 poles (13.2018, -3.1199) (13.5308, -3.1199) (13.8404, -3.6386) (13.8404, -4.1604) knots 0 0 0 1 2 2 2
  spline S227 degree 2 poles (13.4968, -4.7698) (13.5357, -4.671) (13.5681, -4.3663) (13.5681, -4.1604) knots 0 0 0 1 2 2 2
  spline S228 degree 2 poles (13.5681, -4.1604) (13.5681, -3.9546) (13.5357, -3.6515) (13.4951, -3.5494) knots 0 0 0 1 2 2 2
  spline S229 degree 2 poles (13.4951, -3.5494) (13.4546, -3.4473) (13.3136, -3.342) (13.2018, -3.342) knots 0 0 0 1 2 2 2
  spline S230 degree 2 poles (13.2018, -3.342) (13.09, -3.342) (12.9457, -3.4473) (12.9036, -3.5527) knots 0 0 0 1 2 2 2
  spline S231 degree 2 poles (12.9036, -3.5527) (12.863, -3.6548) (12.8339, -3.9659) (12.8339, -4.1621) knots 0 0 0 1 2 2 2
  spline S232 degree 2 poles (12.8339, -4.1621) (12.8339, -4.3728) (12.8598, -4.6548) (12.9019, -4.765) knots 0 0 0 1 2 2 2
  spline S233 degree 2 poles (12.9019, -4.765) (12.9408, -4.8687) (13.0851, -4.9805) (13.2018, -4.9805) knots 0 0 0 1 2 2 2
  spline S234 degree 2 poles (13.2018, -4.9805) (13.312, -4.9805) (13.4562, -4.8752) (13.4968, -4.7698) knots 0 0 0 1 2 2 2
  line L178 (15.2293, -5.1604) -> (14.2536, -5.1604)
  line L179 (14.2536, -5.1604) -> (14.2536, -4.9562)
  line L180 (14.2536, -4.9562) -> (14.6167, -4.9562)
  line L181 (14.6167, -4.9562) -> (14.6167, -3.6159)
  line L182 (14.6167, -3.6159) -> (14.2536, -3.6159)
  line L183 (14.2536, -3.6159) -> (14.2536, -3.4327)
  spline S235 degree 2 poles (14.2536, -3.4327) (14.4595, -3.4327) (14.654, -3.316) (14.6669, -3.154) knots 0 0 0 1 2 2 2
  line L184 (14.6669, -3.154) -> (14.8744, -3.154)
  line L185 (14.8744, -3.154) -> (14.8744, -4.9562)
  line L186 (14.8744, -4.9562) -> (15.2293, -4.9562)
  line L187 (15.2293, -4.9562) -> (15.2293, -5.1604)
  line L188 (16.8533, -3.4603) -> (15.9878, -5.1604)
  line L189 (15.9878, -5.1604) -> (15.7026, -5.1604)
  line L190 (15.7026, -5.1604) -> (16.6167, -3.3954)
  line L191 (16.6167, -3.3954) -> (15.5843, -3.3954)
  line L192 (15.5843, -3.3954) -> (15.5843, -3.1604)
  line L193 (15.5843, -3.1604) -> (16.8533, -3.1604)
  line L194 (16.8533, -3.1604) -> (16.8533, -3.4603)
  point P0 (0, 0)
  point P1 (19.75, 0)
  point P2 (29.6663, 0)
  point P3 (0, 7.25)
  point P4 (0, 8.3891)
  constraints: 4 midpoint, 1 horizontal, 1 horizontal alignment, 1 vertical alignment, 2 other
extrude "Extrusion2" cut sketch "Sketch2" against normal blind 0.4
body "Solid1"
